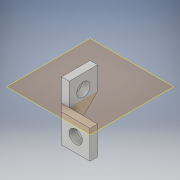
# Autodesk Inventor part: Caixa control - tirador
Saved by Autodesk Inventor 2019 (Build 230136000, 136)
## iProperties
Created: 2018-09-18
Part Number: Caixa control - tirador
Material: Genérico
Document SubType Name: Modeling
Designer: Albert Garangou Culebras
Density: 1 g/cm^3
Appearance: Valor por defecto
Author: Albert Garangou Culebras
Autodesk Inventor part; units mm, degrees
ref_plane "YZ Plane" through (0, 0, 0) normal (1, 0, 0) x (0, 1, 0)
ref_plane "XZ Plane" through (0, 0, 0) normal (0, 1, 0) x (-1, 0, 0)
ref_plane "XY Plane" through (0, 0, 0) normal (0, 0, 1) x (1, 0, 0)
sketch "Boceto2" plane through (0, 0, 0) normal (0, 0, 1) x (1, 0, 0)
  line L0 (0, 0) -> (2, 0)
  line L1 (2, 0) -> (2, -7.5)
  line L2 (2, 0) -> (3, 0)
  line L3 (2.8119, -7.5) -> (0, -7.5)
  line L4 (0, -7.5) -> (0, 0)
  line L5 (3, 0) -> (3, -7.5)
  line L6 (3, -7.5) -> (0, -7.5)
  line L7 (3, 0) -> (6.5, 0)
  line L8 (6.5, 0) -> (8.5, 0)
  line L9 (8.5, 0) -> (8.5, -7.5)
  line L10 (8.5, -7.5) -> (3, -7.5)
  circle A0 centre (5.75, -3.75) radius 1.75
  dimension "d6" = 2
  dimension "d15" = 1
  dimension "d16" = 3.5
  dimension "d17" = 2
  dimension "d18" = 3.5
  constraints: 22 end point, 3 horizontal, 3 perpendicular, 1 centre point, 1 collinear, 1 parallel, 1 point on line, 1 vertical
  measures "d6" distance of L0.start L0.end
  measures "d15" distance of L0.end L2.end
  measures "d16" distance of L2.end L7.end
  measures "d17" distance of L7.end L8.end
  measures "d18" diameter of A0
sketch "Boceto1" plane through (0, 0, 0) normal (1, 0, 0) x (0, 1, 0)
  line L0 (0, 0) -> (0, -2)
  line L1 (0, -2) -> (0, -5.5)
  line L2 (0, -5.5) -> (0, -7.5)
  line L3 (0, -7.5) -> (-2, -7.5)
  line L4 (-2, -7.5) -> (-5.5, -7.5)
  line L5 (0, 0) -> (-5.5, 0)
  line L6 (-5.5, -7.5) -> (-7.5, -7.5)
  line L7 (-7.5, -7.5) -> (-7.5, 0)
  line L8 (-7.5, 0) -> (0, 0)
  dimension "d0" = 2
  dimension "d1" = 3.5
  dimension "d2" = 2
  dimension "d3" = 2
  dimension "d4" = 3.5
  dimension "d5" = 2
  constraints: 18 end point, 3 horizontal, 3 point on line, 1 collinear, 1 perpendicular, 1 vertical
  measures "d0" distance of L0.start L0.end
  measures "d1" distance of L0.end L1.end
  measures "d2" distance of L1.end L2.end
  measures "d3" distance of L2.end L3.end
  measures "d4" distance of L3.end L4.end
  measures "d5" distance of L4.end L6.end
extrude "Extrusión2" add sketch "Boceto2" along normal blind 2
chamfer "Chaflán1" distance 2 angle 45 1 edges at (0, -3.75, 2)
sketch "Boceto4" plane through (0, 0, 2) normal (0, 0, 1) x (1, 0, 0)
  line L0 (8.5, -7.5) -> (9.5, -7.5)
  line L1 (9.5, -7.5) -> (9.5, 0)
  line L2 (9.5, 0) -> (8.5, 0)
  line L3 (8.5, -7.5) -> (8.5, 0) projected
  line L4 (8.5, 0) -> (8.5, -7.5)
  point P0 (0, 0)
  dimension "d24" = 1
  constraints: 8 end point, 2 perpendicular, 1 collinear, 1 horizontal
  measures "d24" distance of L0.start L0.end
extrude "Extrusión3" add sketch "Boceto4" against normal blind 2
ref_plane "Plano de trabajo2" through (0, 0, -7.5) normal (0, 1, 0) x (1, 0, 0)
sketch "Boceto5" plane through (0, 0, -7.5) normal (0, 1, 0) x (1, 0, 0)
  line L0 (0, -7.5) -> (2, -9.5) projected
  line L1 (0, -7.5) -> (2, -7.5)
  line L2 (2, -7.5) -> (2, 0) projected
  line L3 (2, -7.5) -> (2, 0)
  line L4 (0, 0) -> (2, 0) projected
  line L5 (2, 0) -> (0, 0)
  line L6 (2, -7.5) -> (2, -9.5)
  line L7 (0, 0) -> (0, -7.5) projected
  line L8 (0, -7.5) -> (0, 0)
  constraints: 10 end point, 2 vertical, 1 collinear, 1 horizontal, 1 perpendicular
extrude "Extrusión4" add sketch "Boceto5" along normal blind 6
extrude "Extrusión5" cut sketch "Boceto1" along normal blind 2
extrude "Extrusión6" add sketch "Boceto1" along normal blind 2
sketch "Boceto6" plane through (0, -7.5, -7.5) normal (-1, 0, 0) x (0, 0, 1)
  line L0 (0, 13.5) -> (7.5, 13.5) projected
  line L1 (3.75, 13.5) -> (3.75, 11.5)
  line L2 (3.75, 11.5) -> (3.75, 8)
  circle A0 centre (3.75, 9.75) radius 1.75
  point P0 (7.5, 7.5)
  dimension "d33" = 3.5
  constraints: 4 end point, 2 midpoint, 2 vertical, 1 vertical alignment, 2 other
  measures "d33" distance of L1.end L2.end
extrude "Extrusión7" cut sketch "Boceto6" against normal blind 29.5
sketch "Boceto7" plane through (0, 6, -7.5) normal (0, 1, 0) x (1, 0, 0)
  line L0 (0, 0) -> (0, -7.5) projected
  line L1 (0, -7.5) -> (2, -7.5)
  line L2 (2, -9.5) -> (2, 0) projected
  line L3 (2, -7.5) -> (2, -9.5)
  line L4 (0, -7.5) -> (2, -9.5) projected
  line L5 (2, -9.5) -> (0, -7.5)
  constraints: 6 end point, 2 collinear, 1 horizontal
extrude "Extrusión8" cut sketch "Boceto7" against normal blind 6
chamfer "Chaflán2" distance 7.5 angle 45 1 edges at (1, -7.5, -7.5)
